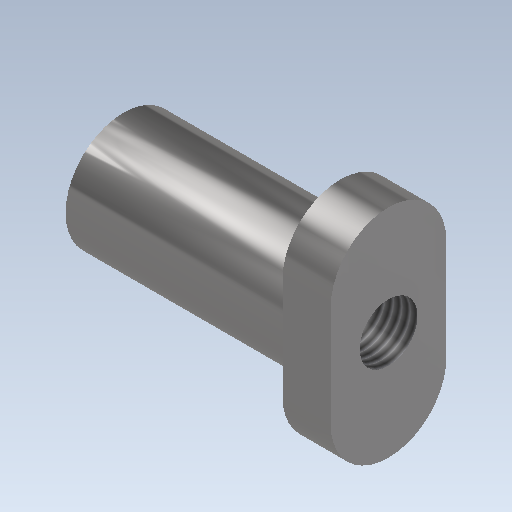
# Autodesk Inventor part: Rotator
Saved by Autodesk Inventor 2021.3 (Build 253353000, 353)
## iProperties
Created: 2021-06-01
Part Number: Rotator
Material: Steel, Alloy
Document SubType Name: Modeling
Designer: vivek
Density: 7.85 g/cm^3
Appearance: Semi-Polished
Author: vivek
Autodesk Inventor part; units mm, degrees
ref_plane "YZ Plane" through (0, 0, 0) normal (1, 0, 0) x (0, 1, 0)
ref_plane "XZ Plane" through (0, 0, 0) normal (0, 1, 0) x (-1, 0, 0)
ref_plane "XY Plane" through (0, 0, 0) normal (0, 0, 1) x (1, 0, 0)
sketch "Sketch1" plane through (0, 0, 0) normal (1, 0, 0) x (0, 1, 0)
  circle A0 centre (0, 0) radius 6
  circle A1 centre (0, 0) radius 12
  dimension "d0" = 12
  dimension "d1" = 24
  constraints: 2 centre point, 2 coincident
  measures "d0" diameter of A0
  measures "d1" diameter of A1
extrude "Extrusion1" add sketch "Sketch1" along normal blind 45
sketch "Sketch2" plane through (45, 0, 0) normal (1, 0, 0) x (0, 0, -1)
  circle A0 centre (0, 0) radius 6 projected
  circle A1 centre (0, 0) radius 12 projected
  line L0 (12, -22.5) -> (-12, -22.5)
  line L1 (-12, -22.5) -> (-12, 22.5)
  line L2 (-12, 22.5) -> (12, 22.5)
  line L3 (12, 22.5) -> (12, -22.5)
  line L4 (0, 0) -> (3.4418, 0)
  point P0 (12, 0)
  dimension "d4" = 45
  constraints: 10 end point, 2 parallel, 2 perpendicular, 2 tangent, 1 horizontal, 1 midpoint, 1 point on line
  measures "d4" distance of L0.end L1.end
extrude "Extrusion2" add sketch "Sketch2" along normal blind 10
fillet "Fillet1" radius 12 4 edges at (50, -22.5, -12) (50, -22.5, 12) (50, 22.5, -12) (50, 22.5, 12)
thread "Thread1" size "M12x1.75" class "6H" standard "ANSI Metric M Profile" full length
body "Solid1"
